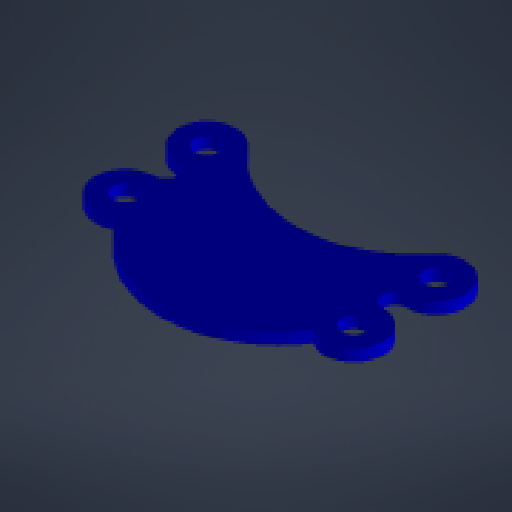
# Autodesk Inventor part: ts_holder
Saved by Autodesk Inventor 2024 (Build 280153000, 153)
## iProperties
Created: 2023-05-15
Part Number: ts_holder
Material: Типовые
Document SubType Name: Modeling
Designer: user
Density: 1 g/cm^3
Appearance: По умолчанию
Author: user
Autodesk Inventor part; units mm, degrees
ref_plane "YZ Plane" through (0, 0, 0) normal (1, 0, 0) x (0, 1, 0)
ref_plane "XZ Plane" through (0, 0, 0) normal (0, 1, 0) x (-1, 0, 0)
ref_plane "XY Plane" through (0, 0, 0) normal (0, 0, 1) x (1, 0, 0)
sketch "Эскиз1" plane through (0, 0, 0) normal (0, 0, 1) x (1, 0, 0)
  circle A0 centre (0, 0) radius 2 projected
  circle A1 centre (-39, -14) radius 2 projected
  circle A2 centre (-39, 0) radius 2 projected
  circle A3 centre (0, -14) radius 2 projected
  arc A4 (-35.1, 3.1289) -> (-39, -5) centre (-39, 0) ccw
  arc A5 (-39, -9) -> (-36.2789, -18.1947) centre (-39, -14) ccw
  arc A6 (0, -5) -> (-3.9, 3.1289) centre (0, 0) ccw
  arc A7 (-2.7211, -18.1947) -> (0, -9) centre (0, -14) ccw
  arc A8 (-35.1, 3.1289) -> (-3.9, 3.1289) centre (-19.5, 15.6445) ccw
  arc A9 (-36.2789, -18.1947) -> (-2.7211, -18.1947) centre (-19.5, -7.3105) ccw
  arc A10 (0, -5) -> (0, -9) centre (0, -7) ccw
  arc A11 (-39, -9) -> (-39, -5) centre (-39, -7) ccw
  point P0 (0, 0)
  dimension "d0" = 2
  dimension "d1" = 5
  dimension "d2" = 20
  dimension "d3" = 20
  constraints: 16 point on circle, 8 centre point, 6 tangent, 4 coincident, 4 equal radius, 2 other
  measures "d0" radius of A11
  measures "d1" radius of A5
  measures "d2" radius of A8
  measures "d3" radius of A9
extrude "Выдавливание1" add sketch "Эскиз1" along normal blind 2
